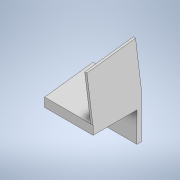
# Autodesk Inventor part: 斜面
Saved by Autodesk Inventor 2020 (Build 240168000, 168)
## iProperties
Created: 2020-12-07
Part Number: 斜面
Material: 常规
Document SubType Name: Sheet Metal
Designer: huang
Density: 1 g/cm^3
Sheet Metal Rule: 默认_mm
Appearance: 默认
Author: huang
## iProperties of the stored document _3D 打印.ipt
Created: 2020-12-11
Part Number: _3D 打印
Material: 常规
Document SubType Name: Modeling
Designer: huang
Density: 1 g/cm^3
Appearance: 默认
Author: huang
Autodesk Inventor part; units mm, degrees
ref_plane "YZ Plane" through (0, 0, 0) normal (1, 0, 0) x (0, 1, 0)
ref_plane "XZ Plane" through (0, 0, 0) normal (0, 1, 0) x (-1, 0, 0)
ref_plane "XY Plane" through (0, 0, 0) normal (0, 0, 1) x (1, 0, 0)
sketch "草图1" plane through (0, 0, 0) normal (0, 1, 0) x (-1, 0, 0)
  line L0 (0, 0) -> (65, 0)
  line L1 (65, 0) -> (65, -65)
  line L2 (65, -65) -> (0, -65)
  line L3 (0, -65) -> (0, 0)
  dimension "d0" = 65
  dimension "d1" = 65
  constraints: 8 end point, 2 parallel, 1 horizontal, 1 perpendicular
  measures "d0" distance of L0.end L1.end
  measures "d1" distance of L1.end L2.end
extrude "拉伸1" add sketch "草图1" along normal blind 10
chamfer "倒角1" distance 65 angle 7 1 edges at (-32.5, 10, 0) measured on face at (-32.5, 10, -0.5)
sketch "草图2" plane through (0, 0, 0) normal (0, -1, 0) x (1, 0, 0)
  line L0 (-65, 0) -> (0, 0) projected
  line L1 (-32.5, 0) -> (-32.5, -65)
  line L2 (0, -65) -> (-65, -65) projected
  circle A0 centre (-32.5, -32.5) radius 1.95
  dimension "d7" = 3.9
  constraints: 3 midpoint, 2 end point, 1 centre point
  measures "d7" diameter of A0
extrude "拉伸2" cut sketch "草图2" against normal blind 4
sketch "草图3" plane through (0, 0, 0) normal (0, -1, 0) x (1, 0, 0)
  line L0 (0, -65) -> (-65, -65) projected
  line L1 (-65, -65) -> (-65, 0) projected
  line L2 (0, -65) -> (-65, -65)
  line L3 (-65, -65) -> (-65, -59)
  line L4 (-65, -59) -> (0, -59)
  line L5 (0, -59) -> (0, -65)
  point P0 (0, 0)
  dimension "d10" = 6
  constraints: 8 end point, 2 parallel, 1 horizontal, 1 perpendicular, 1 point on line
  measures "d10" distance between parallel lines of L0 L4
extrude "拉伸3" add sketch "草图3" along normal blind 50
sketch "草图4" plane through (-65, 10, -65) normal (0, 0.9925462, 0.1218693) x (1, 0, 0)
  line L0 (65, -7.3122) -> (65, 0) projected
  line L1 (65, 0) -> (62, 0)
  line L2 (62, 0) -> (62, -65.7342)
  line L3 (62, -65.7342) -> (65, -65.7342)
  line L4 (65, -65.7342) -> (65, 0)
  dimension "d13" = 3
  constraints: 8 end point, 2 parallel, 1 horizontal, 1 perpendicular
  measures "d13" distance between parallel lines of L2 L4
extrude "拉伸4" add sketch "草图4" along normal blind 65
sketch "草图5" plane through (0, 0, 0) normal (0, -1, 0) x (1, 0, 0)
  line L0 (-65, -59) -> (-65, -65) projected
  line L1 (0, 0) -> (-65, 0)
  line L2 (-65, 0) -> (-65, -59)
  line L3 (-65, -59) -> (0, -59)
  line L4 (0, -59) -> (0, 0)
  constraints: 8 end point, 2 parallel, 1 horizontal, 1 perpendicular
extrude "拉伸5" add sketch "草图5" along normal blind 10
sketch "草图6" plane through (0, -10, 0) normal (0, -1, 0) x (1, 0, 0)
  circle A0 centre (-32.5, -32.5) radius 1.95 projected
  circle A1 centre (-32.5, -32.5) radius 2.5
  point P0 (0, 0)
  dimension "d18" = 5
  constraints: 1 centre point, 1 coincident
  measures "d18" diameter of A1
extrude "拉伸6" cut sketch "草图6" against normal blind 13 contours A0 | A1
equation "\"折弯半径\" = 厚度"
equation "\"折弯释压宽度\" = 厚度"
equation "\"折弯释压深度\" = 0.5 * 厚度"
equation "\"拐角释压尺寸\" = 4 * 厚度"
equation "\"最小余量\" = 2 * 厚度"
equation "\"过渡半径\" = 折弯半径"
equation "\"Jacobi半径尺寸\" = 折弯半径"
equation "\"间隙大小\" = 厚度"
equation "\"厚度\" = 0.5"
